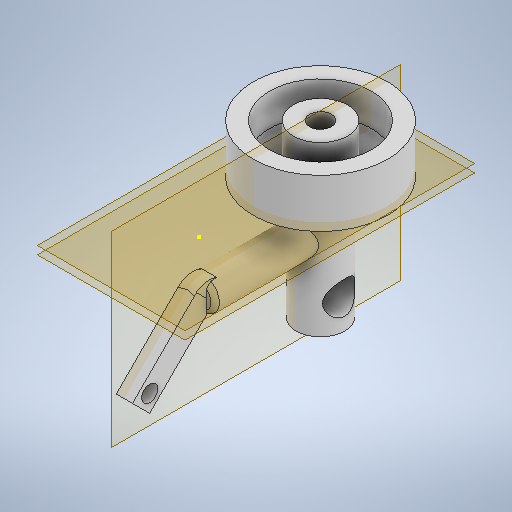
# Autodesk Inventor part: WHEELS
Saved by Autodesk Inventor 2025 (Build 290162010, 162A)
## iProperties
Created: 2024-07-31
Part Number: WHEELS
Material: Generic
Document SubType Name: Modeling
Designer: darkb
Density: 1 g/cm^3
Appearance: Default
Author: darkb
Autodesk Inventor part; units mm, degrees
ref_plane "XY Plane" through (0, 0, 0) normal (0, 0, 1) x (1, 0, 0)
sketch "Sketch1" plane through (0, 0, 0) normal (0, 1, 0) x (-1, 0, 0)
  circle A0 centre (0, 0) radius 9.248617
  circle A1 centre (0, 0) radius 2.97815
  dimension "d0" = 5.9563
  constraints: 2 centre point, 2 coincident
  measures "d0" diameter of A1
extrude "Extrusion1" add sketch "Sketch1" along normal blind 6.35
shell "Shell1" thickness 2.54 both sides yes removed faces 1 at (-7.040032, 6.35, -0.975352)
sketch "Sketch2" plane through (0, -1.27, 0) normal (0, -1, 0) x (1, 0, 0)
  circle A0 centre (0, 0) radius 3.81
  dimension "d4" = 7.62
  constraints: 1 centre point, 1 coincident
  measures "d4" diameter of A0
extrude "Extrusion2" add sketch "Sketch2" along normal blind 19.05
sketch "Sketch3" plane through (0, -20.32, 0) normal (0, -1, 0) x (1, 0, 0)
  point P0 (0, 0)
sketch "Sketch4" plane through (0, 0, 0) normal (1, 0, 0) x (0, 1, 0)
  circle A0 centre (-15.774432, 0) radius 2.54
  point P0 (0, 0)
  dimension "d7" = 5.08
  constraints: 1 centre point
  measures "d7" diameter of A0
extrude "Extrusion3" cut sketch "Sketch4" along normal blind 19.05 and the other way blind 9.525
sketch "Sketch5" plane through (0, 0, 0) normal (0, 0, 1) x (1, 0, 0)
  point P0 (0, 0)
sketch "Sketch6" plane through (0, 0, 0) normal (0, 0, 1) x (1, 0, 0)
  circle A0 centre (0, -7.888733) radius 2.54
  point P0 (0, 0)
  dimension "d12" = 5.08
  constraints: 1 centre point
  measures "d12" diameter of A0
extrude "Extrusion4" add sketch "Sketch6" along normal blind 19.05
chamfer "Chamfer1" distance 0.6731 angle 45 1 edges at (-2.54, -7.8887, 19.05)
sketch "Sketch7" plane through (0, -7.888733, 19.05) normal (0, 0, 1) x (1, 0, 0)
  point P0 (0, 7.888733)
sketch "Sketch8" plane through (0, -7.888733, 19.05) normal (0, 0, 1) x (1, 0, 0)
  point P0 (0, 7.888733)
sketch "Sketch9" plane through (0, 0, 0) normal (1, 0, 0) x (0, 1, 0)
  line L0 (-10.428733, 3.81) -> (-10.428733, 18.3769)
  line L1 (-9.755633, 19.05) -> (-6.021833, 19.05)
  line L2 (-10.428733, 18.3769) -> (-9.755633, 19.05)
  line L3 (-9.755633, 19.05) -> (-18.735889, 28.030256)
  line L4 (-18.735889, 28.030256) -> (-16.041813, 30.724333)
  line L5 (-16.041813, 30.724333) -> (-6.021833, 20.704354)
  line L6 (-6.021833, 20.704354) -> (-8.71591, 18.010277)
  line L7 (-8.71591, 18.010277) -> (-10.428733, 19.7231)
  point P0 (0, 0)
  point P1 (-7.676187, 19.05)
  dimension "d18" = 12.7
  dimension "d19" = 3.81
  constraints: 12 end point, 3 perpendicular, 2 point on line
  measures "d18" distance of L1.start L3.end
  measures "d19" distance of L3.end L4.end
extrude "Extrusion5" add sketch "Sketch9" along normal mid plane 2.54 contours L3 L4 L5 L6 L1
sketch "Sketch10" plane through (-1.27, -16.041813, 30.724333) normal (0, 0.7071068, 0.7071068) x (1, 0, 0)
  line L0 (0, 14.170391) -> (2.54, 14.170391)
  line L1 (0, 14.170391) -> (2.463002, 14.170391)
  line L2 (2.463002, 14.170391) -> (2.463002, 16.754206)
  line L3 (2.463002, 16.754206) -> (0, 16.754206)
  line L4 (0, 16.754206) -> (0, 14.170391)
  point P0 (1.27, 33.068659)
  dimension "d22" = 2.58381
  constraints: 8 end point, 2 parallel, 1 horizontal, 1 perpendicular
  measures "d22" distance of L3.end L0.start
extrude "Extrusion6" add sketch "Sketch10" against normal blind 2.54
fillet "Fillet1" radius 3.175 1 edges at (-0.0385, -4.1948, 18.8773)
sketch "Sketch11" plane through (-1.27, 0, 0) normal (-1, 0, 0) x (0, 0, 1)
  point P0 (0, 0)
sketch "Sketch12" plane through (-1.27, 0, 0) normal (-1, 0, 0) x (0, 0, 1)
  circle A0 centre (28.030256, -16.041813) radius 1.27
  point P0 (0, 0)
  dimension "d26" = 2.54
  constraints: 1 centre point
  measures "d26" diameter of A0
extrude "Extrusion7" cut sketch "Sketch12" against normal blind 2.54
ref_plane "Work Plane1" through (0, -1.27, 0) normal (0, 1, 0) x (-1, 0, 0)
split_face "Split1"
body "Solid1"
